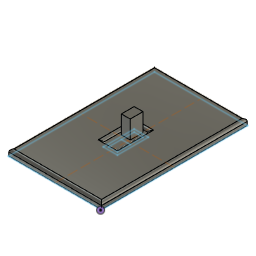
light switch v3 (Autodesk Fusion 360 design; units mm, degrees)
Autodesk Fusion 360 part; units mm, degrees
sketch "Sketch1" plane through (0, 0, 0) normal (0, 0, 1) x (1, 0, 0)
  line L0 (-69.9882, 110.6753) -> (0.0118, 110.6753)
  line L1 (0.0118, 110.6753) -> (0.0118, 0.6753)
  line L2 (0.0118, 0.6753) -> (-69.9882, 0.6753)
  line L3 (-69.9882, 0.6753) -> (-69.9882, 110.6753)
  line L4 (-34.9882, 0.6753) -> (-34.9882, 110.6753) construction
  line L5 (0.0118, 55.6753) -> (-69.9882, 55.6753) construction
  line L6 (-34.9882, 65.6753) -> (-29.6482, 65.6753)
  line L7 (-34.9882, 65.6753) -> (-40.3282, 65.6753)
  line L8 (-40.3282, 65.6753) -> (-40.3282, 42.3553)
  line L9 (-40.3282, 42.3553) -> (-29.6482, 42.3553)
  line L10 (-29.6482, 42.3553) -> (-29.6482, 65.6753)
  line L11 (-34.9882, 63.6753) -> (-31.6482, 63.6753)
  line L12 (-31.6482, 44.3553) -> (-31.6482, 63.6753)
  line L13 (-38.3282, 44.3553) -> (-31.6482, 44.3553)
  line L14 (-38.3282, 63.6753) -> (-38.3282, 44.3553)
  line L15 (-34.9882, 63.6753) -> (-38.3282, 63.6753)
  line L16 (-38.3282, 54.0153) -> (-31.6482, 54.0153)
  dimension "d10" = 70
  dimension "d11" = 110
  dimension "d31" = 45
  dimension "d35" = 5.34
  dimension "d36" = 5.34
  dimension "d37" = 23.32
  dimension "d38" = 10.68
  dimension "d39" = -2
  constraint horizontal L0
  constraint vertical L1
  constraint horizontal L2
  constraint vertical L3
  constraint midpoint L2 L4.start
  constraint midpoint L0 L4.end
  constraint midpoint L1 L5.start
  constraint midpoint L3 L5.end
  constraint perpendicular L4 L6
  constraint perpendicular L4 L7
  constraint perpendicular L7 L8
  constraint perpendicular L4 L9
  constraint midpoint L14 L16.start
  constraint midpoint L12 L16.end
  measures "d10" distance of L0.start L0.end
  measures "d11" distance of L0.start L2.end
  measures "d31" distance of L4.end L6.start
  measures "d35" distance of L6.start L6.end
  measures "d36" distance of L6.start L7.end
  measures "d37" distance of L7.end L8.end
  measures "d38" distance of L8.end L9.end
extrude "Extrude4" add sketch "Sketch1" along normal blind 4.63 contours L0 L1 L2 L3
extrude "Extrude5" add sketch "Sketch1" along normal blind 3 contours L6 L7 L8 L9 L10
extrude "Extrude6" add sketch "Sketch1" along normal blind 16.71 contours L11 L12 L14 L15 L16
extrude "Extrude7" add sketch "Sketch1" along normal blind 3 contours L12 L13 L14 L16
fillet "Fillet1" radius 2 4 edges at (0.0118, 55.6753, 4.63) (-34.9882, 0.6753, 4.63) (-69.9882, 55.6753, 4.63) (-34.9882, 110.6753, 4.63)
fillet "Fillet2" radius 2 4 edges at (-40.3282, 54.0153, 4.63) (-34.9882, 65.6753, 4.63) (-29.6482, 54.0153, 4.63) (-34.9882, 42.3553, 4.63)
extrude "Extrude2" [suppressed]
extrude "Extrude1" [suppressed]
extrude "Extrude3" [suppressed]
sketch "Sketch2" plane through (0, 0, 0) normal (1, 0, 0) x (0, 1, 0)
equation "overall_length = 110 mm"
equation "overall_width = 70 mm"
equation "switch_width = 8.95 mm"
equation "switch_protrusion = 16.71 mm"
equation "switch_height = 18.15 mm"
equation "switch_housing_height = 23.32 mm"
equation "switch_housing_width = 10.68 mm"
equation "centering = 29.5 mm"
equation "overall_height_protrusion = 4.63 mm"
equation "d10 = overall_width"
equation "d11 = overall_length"
equation "centering_fromtop = 45 mm"
equation "d31 = centering_fromtop"
equation "d35 = switch_housing_width / 2"
equation "d36 = switch_housing_width / 2"
equation "d37 = switch_housing_height"
equation "d38 = switch_housing_width"
equation "d40 = switch_protrusion"
equation "d42 = overall_height_protrusion"
equation "d44 = overall_height_protrusion - 1 mm"
equation "d46 = overall_height_protrusion"
equation "d50 = switch_protrusion"
